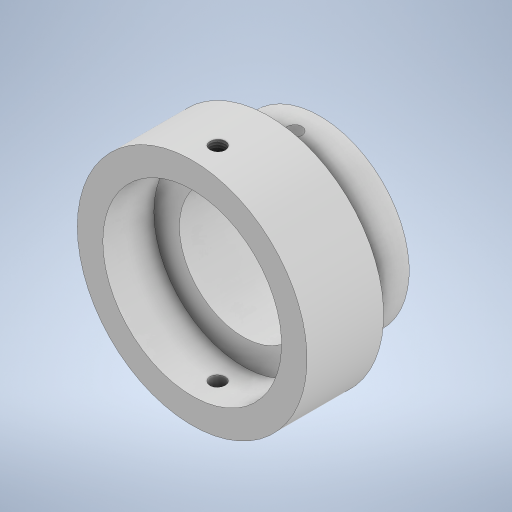
# Autodesk Inventor part: Муфта штурвал, вал 25
Saved by Autodesk Inventor 2023 (Build 270158000, 158)
## iProperties
Created: 2022-05-21
Part Number: Муфта штурвал, вал 25
Material: Типовые
Document SubType Name: Modeling
Designer: avkap
Density: 1 g/cm^3
Appearance: По умолчанию
Author: avkap
Autodesk Inventor part; units mm, degrees
ref_plane "YZ Plane" through (0, 0, 0) normal (1, 0, 0) x (0, 1, 0)
ref_plane "XZ Plane" through (0, 0, 0) normal (0, 1, 0) x (-1, 0, 0)
ref_plane "XY Plane" through (0, 0, 0) normal (0, 0, 1) x (1, 0, 0)
sketch "Эскиз1" plane through (0, 0, 0) normal (0, 1, 0) x (-1, 0, 0)
  line L0 (17.5, -40) -> (17.5, -50)
  line L1 (17.5, -50) -> (12.5, -50)
  line L2 (12.5, -50) -> (12.5, -65)
  line L3 (12.5, -65) -> (17.5, -65)
  line L4 (22.5, -55) -> (22.5, -40)
  line L5 (22.5, -40) -> (17.5, -40)
  line L6 (12.5, -65) -> (17.5, -65)
  line L7 (22.5, -50) -> (22.5, -55)
  line L8 (22.5, -55) -> (17.5, -55)
  line L9 (17.5, -55) -> (17.5, -65)
  line L10 (12.5, -65) -> (0, -65)
  line L11 (0, -65) -> (0, -40)
  line L12 (17.5, -40) -> (0, -40)
  dimension "d21" = 10
  dimension "d22" = 15
  dimension "d23" = 5
  dimension "d24" = 5
  dimension "d26" = 12.5
  dimension "d39" = 17.5
  dimension "d40" = 5
  constraints: 26 end point, 8 perpendicular, 2 horizontal, 2 point on line
  measures "d21" distance of L0.start L0.end
  measures "d22" distance of L1.end L2.end
  measures "d23" distance of L3.end L2.end
  measures "d24" distance of L4.start L7.start
  measures "d26" distance of L2.end L10.end
  measures "d39" distance of L0.start L11.end
  measures "d40" distance of L4.end L0.start
revolve "Вращение1" add sketch "Эскиз1" angle 360 about axis through (0, 0, -65) along (0, 0, 1) contours L5 L4 L8 L9 L3 L2 L1 L0
sketch "Эскиз4" plane through (0, 0, 0) normal (0, 1, 0) x (-1, 0, 0)
  line L0 (12.5, -65) -> (-12.5, -65) projected
  line L1 (0, -65) -> (0, -60)
  line L2 (17.5, -40) -> (-17.5, -40) projected
  line L3 (0, -40) -> (0, -45)
  circle A0 centre (0, -60) radius 1.5
  circle A1 centre (0, -45) radius 1.5
  point P0 (0, 0)
  dimension "d27" = 5
  dimension "d28" = 5
  dimension "d29" = 3
  dimension "d30" = 3
  constraints: 4 end point, 2 centre point, 2 coincident, 2 midpoint, 1 point on line, 1 vertical
  measures "d27" distance of L1.start L1.end
  measures "d28" distance of L3.start L3.end
  measures "d29" diameter of A0
  measures "d30" diameter of A1
extrude "Выдавливание3" cut sketch "Эскиз4" along normal blind 49.75 and the other way blind 43
thread "Резьба1" size "M3x0.5" class "6H" standard "ANSI Metric M Profile" length 15
thread "Резьба2" size "M3x0.5" class "6H" standard "ANSI Metric M Profile" length 15
